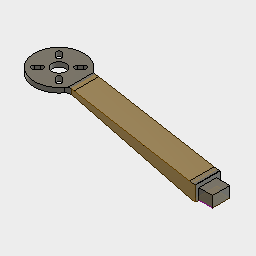
Motor Arm V1.2 v1 (Autodesk Fusion 360 design; units mm, degrees)
Autodesk Fusion 360 part; units mm, degrees
sketch "Sketch1" plane through (0, 0, 0) normal (1, 0, 0) x (0, 0, -1)
  line L0 (-21.2104, 3.553) -> (-6.2104, 3.553)
  line L1 (-6.2104, 3.553) -> (-6.2104, 12.553)
  line L2 (-6.2104, 12.553) -> (-21.2104, 12.553)
  line L3 (-21.2104, 12.553) -> (-21.2104, 3.553)
  dimension "d1" = 15
  dimension "d2" = 9
  constraint horizontal L0
  constraint vertical L1
  constraint horizontal L2
  constraint vertical L3
extrude "Extrude1" add sketch "Sketch1" along normal blind 2
sketch "Sketch2" plane through (2, 0, 0) normal (1, 0, 0) x (0, 0, -1)
  line L0 (-21.2104, 12.553) -> (-21.2104, 3.553)
  line L1 (-21.2104, 3.553) -> (-6.2104, 3.553)
  line L2 (-6.2104, 3.553) -> (-6.2104, 12.553)
  line L3 (-6.2104, 12.553) -> (-21.2104, 12.553)
  line L4 (-19.1104, 5.653) -> (-8.3104, 5.653)
  line L5 (-8.3104, 5.653) -> (-8.3104, 10.453)
  line L6 (-8.3104, 10.453) -> (-19.1104, 10.453)
  line L7 (-19.1104, 10.453) -> (-19.1104, 5.653)
  dimension "d5" = 2.1
sketch "Sketch4" plane through (0, 0, 21.2104) normal (0, 0, 1) x (1, 0, 0)
  line L0 (0, 12.553) -> (0, 3.553)
  line L1 (0, 3.553) -> (2, 3.553)
  line L2 (2, 3.553) -> (2, 12.553)
  line L3 (2, 12.553) -> (0, 12.553)
  line L4 (0, 12.553) -> (-73.8606, 25.5766)
  line L5 (-73.8606, 25.5766) -> (-73.8606, 22.5766)
  line L6 (-73.8606, 22.5766) -> (0, 3.553)
  dimension "d12" = 75
  dimension "d22" = 3
  constraint vertical L5
  measures "d12" distance of origin
  measures "d22" distance of origin
sketch "Sketch5" plane through (2, 0, 0) normal (1, 0, 0) x (0, 0, -1)
  line L0 (-21.2104, 12.553) -> (-21.2104, 3.553)
  line L1 (-21.2104, 3.553) -> (-6.2104, 3.553)
  line L2 (-6.2104, 3.553) -> (-6.2104, 12.553)
  line L3 (-6.2104, 12.553) -> (-21.2104, 12.553)
  line L4 (-21.2104, 3.553) -> (-6.2104, 3.553)
  line L5 (-6.2104, 3.553) -> (-6.2104, 5.553)
  line L6 (-6.2104, 5.553) -> (-21.2104, 5.553)
  line L7 (-21.2104, 5.553) -> (-21.2104, 3.553)
  constraint horizontal L4
  constraint vertical L5
  constraint horizontal L6
  constraint vertical L7
  constraint coincident L2
sketch "Sketch7" plane through (2, 0, 0) normal (1, 0, 0) x (0, 0, -1)
  line L0 (-21.2104, 12.553) -> (-21.2104, 3.553)
  line L1 (-21.2104, 3.553) -> (-6.2104, 3.553)
  line L2 (-6.2104, 3.553) -> (-6.2104, 12.553)
  line L3 (-6.2104, 12.553) -> (-21.2104, 12.553)
  line L4 (-8.6104, 5.553) -> (-8.6104, 3.553)
  line L5 (-8.6104, 3.553) -> (-19.2104, 3.553)
  line L6 (-8.6104, 5.553) -> (-8.6104, 10.153)
  line L7 (-8.6104, 10.153) -> (-19.2104, 10.153)
  line L8 (-19.2104, 3.553) -> (-19.2104, 10.153)
  dimension "d48" = 10.6
  dimension "d49" = 6.6
  constraint coincident L1 origin
  constraint perpendicular L1 L4
  constraint parallel L2 L6
  constraint parallel L3 L7
  constraint perpendicular L7 L8
  measures "d49" distance of origin
extrude "Extrude6" add sketch "Sketch7" along normal blind 8.3 contours L1 L4 L5 L6 L7 L8
sketch "Sketch8" plane through (0, 3.553, 0) normal (0, -1, 0) x (1, 0, 0)
  line L0 (0, 21.2104) -> (0, 6.2104)
  line L1 (0, 6.2104) -> (2, 6.2104)
  line L2 (2, 6.2104) -> (2, 8.6104)
  line L3 (2, 8.6104) -> (10.3, 8.6104)
  line L4 (10.3, 8.6104) -> (10.3, 19.2104)
  line L5 (2, 19.2104) -> (2, 21.2104)
  line L6 (2, 21.2104) -> (0, 21.2104)
  line L7 (10.3, 19.2104) -> (2, 19.2104)
extrude "Extrude7" add sketch "Sketch4" against normal blind 15 contours L0 L4 L5 L6
sketch "Sketch9" plane through (2.1467, 12.1745, 0) normal (0.173648, 0.984808, 0) x (0, 0, -1)
  line L0 (-21.2104, 77.1798) -> (-21.2104, 2.1798)
  line L1 (-21.2104, 2.1798) -> (-6.2104, 2.1798)
  line L2 (-6.2104, 2.1798) -> (-6.2104, 77.1798)
  line L3 (-6.2104, 77.1798) -> (-21.2104, 77.1798)
sketch "Sketch10" plane through (0, 0, 21.2104) normal (0, 0, 1) x (1, 0, 0)
  line L0 (0, 3.553) -> (2, 3.553)
  line L1 (2, 3.553) -> (2, 12.553)
  line L2 (2, 12.553) -> (0, 12.553)
  line L3 (0, 12.553) -> (-73.8606, 25.5766)
  line L4 (-73.8606, 25.5766) -> (-73.8606, 22.5766)
  line L5 (-73.8606, 22.5766) -> (0, 3.553)
sketch "Sketch11" plane through (-73.8606, 0, 0) normal (-1, 0, 0) x (0, 0, 1)
  line L0 (21.2104, 22.5766) -> (21.2104, 25.5766)
  line L1 (21.2104, 25.5766) -> (6.2104, 25.5766)
  line L2 (6.2104, 25.5766) -> (6.2104, 22.5766)
  line L3 (6.2104, 22.5766) -> (21.2104, 22.5766)
  line L4 (6.2104, 25.5766) -> (21.2104, 25.5766)
  line L5 (21.2104, 25.5766) -> (21.2104, 22.5766)
  line L6 (21.2104, 22.5766) -> (6.2104, 22.5766)
  line L7 (6.2104, 22.5766) -> (6.2104, 25.5766)
  constraint horizontal L4
  constraint vertical L5
  constraint horizontal L6
  constraint vertical L7
extrude "Extrude8" add sketch "Sketch11" along normal blind 2
sketch "Sketch12" plane through (0, 25.5766, 0) normal (0, 1, 0) x (-1, 0, 0)
  line L0 (73.8606, 21.2104) -> (73.8606, 6.2104)
  line L1 (73.8606, 6.2104) -> (75.8606, 6.2104)
  line L2 (75.8606, 6.2104) -> (75.8606, 21.2104)
  line L3 (75.8606, 21.2104) -> (73.8606, 21.2104)
  circle A0 centre (88.8606, 13.7104) radius 15
extrude "Extrude9" add sketch "Sketch12" against normal blind 3 contours L2 A0 picked at (89.1298, 18.4664)
sketch "Sketch13" plane through (0, 25.5766, 0) normal (0, 1, 0) x (-1, 0, 0)
  line L0 (73.8606, 21.2104) -> (73.8606, 6.2104)
  line L1 (73.8606, 6.2104) -> (75.8606, 6.2104)
  line L2 (75.8606, 6.2104) -> (75.8606, 6.2271)
  arc A0 (75.8606, 6.2271) -> (75.8606, 21.1937) centre (88.8606, 13.7104) ccw
  line L3 (75.8606, 21.1937) -> (75.8606, 21.2104)
  line L4 (75.8606, 21.2104) -> (73.8606, 21.2104)
  circle A1 centre (88.8606, 13.7104) radius 4.3
  line L5 (85.82, 10.6699) -> (87.82, 10.6699) construction
  line L6 (82.1431, 9.2557) -> (80.1632, 7.2758)
  arc A2 (80.1632, 7.2758) -> (82.4259, 5.013) centre (81.2945, 6.1444) ccw
  line L7 (82.4259, 5.013) -> (84.4058, 6.9929)
  arc A3 (84.4058, 6.9929) -> (82.1431, 9.2557) centre (83.2744, 8.1243) ccw
  line L8 (84.4058, 9.2557) -> (80.1632, 5.013) construction
  line L9 (93.3154, 9.2557) -> (97.558, 5.013) construction
  arc A4 (95.2953, 5.013) -> (97.558, 7.2758) centre (96.4266, 6.1444) ccw
  line L10 (97.558, 7.2758) -> (95.5781, 9.2557)
  line L11 (93.3154, 6.9929) -> (95.2953, 5.013)
  arc A5 (95.5781, 9.2557) -> (93.3154, 6.9929) centre (94.4467, 8.1243) ccw
  line L12 (93.3154, 18.1652) -> (97.558, 22.4078) construction
  arc A6 (97.558, 20.1451) -> (95.2953, 22.4078) centre (96.4266, 21.2765) ccw
  line L13 (95.2953, 22.4078) -> (93.3154, 20.4279)
  line L14 (95.5781, 18.1652) -> (97.558, 20.1451)
  arc A7 (93.3154, 20.4279) -> (95.5781, 18.1652) centre (94.4467, 19.2966) ccw
  line L15 (84.4058, 18.1652) -> (80.1632, 22.4078) construction
  arc A8 (82.4259, 22.4078) -> (80.1632, 20.1451) centre (81.2945, 21.2765) ccw
  line L16 (80.1632, 20.1451) -> (82.1431, 18.1652)
  line L17 (84.4058, 20.4279) -> (82.4259, 22.4078)
  arc A9 (82.1431, 18.1652) -> (84.4058, 20.4279) centre (83.2744, 19.2966) ccw
  dimension "d32" = 8.6
  dimension "d53" = 2
  dimension "d54" = 3.2
  dimension "d56" = 360
  constraint concentric A0 A1
  constraint coincident A1 origin
  constraint horizontal L5
  constraint tangent L6 A2
  constraint tangent A2 L7
  constraint parallel L6 L7
  constraint tangent L7 A3
  constraint tangent L6 A3
  constraint midpoint A3
  constraint midpoint A2 origin
  measures "d32" diameter of A1
  measures "d53" distance of origin
  measures "d54" diameter of A2
extrude "Extrude10" cut sketch "Sketch13" against normal blind 3 contours A1
sketch "Sketch14" plane through (0, 22.5766, 0) normal (0, -1, 0) x (1, 0, 0)
  circle A0 centre (-88.8606, 13.7104) radius 4.3
  line L0 (-73.8606, 6.2104) -> (-73.8606, 21.2104)
  line L1 (-73.8606, 21.2104) -> (-75.8606, 21.2104)
  line L2 (-75.8606, 21.2104) -> (-75.8606, 21.1937)
  arc A1 (-75.8606, 21.1937) -> (-75.8606, 6.2271) centre (-88.8606, 13.7104) ccw
  line L3 (-75.8606, 6.2271) -> (-75.8606, 6.2104)
  line L4 (-75.8606, 6.2104) -> (-73.8606, 6.2104)
  arc A2 (-73.8606, 6.2104) -> (-77.0082, 4.5169) centre (-73.8606, 2.4386) ccw
  line L5 (-73.8606, 13.7104) -> (-77.6606, 13.7117)
  arc A3 (-77.0018, 22.9062) -> (-73.8554, 21.2104) centre (-73.8528, 24.9823) ccw
  constraint tangent L4 A2
  constraint coincident A1 origin
  constraint midpoint L0
extrude "Extrude11" add sketch "Sketch14" against normal blind 3 contours A1 L3 L4 A2 | L1 L2 A1 A3
fillet "Fillet1" radius 20 1 edges at (-73.8606, 22.5766, 13.7104)
fillet "Fillet2" radius 20 1 edges at (-73.8606, 25.5766, 13.7104)
fillet "Fillet3" radius 20 1 edges at (0, 12.553, 13.7104)
extrude "Extrude12" cut sketch "Sketch13" against normal blind 3 contours A1 | L6 A2 L7 A3 | A4 L10 L11 A5 | A6 L13 L14 A7 | A8 L16 L17 A9
